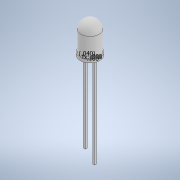
# Autodesk Inventor part: LED
Saved by Autodesk Inventor 2022 (Build 260153000, 153)
## iProperties
Created: 2022-10-09
Part Number: LED
Material: Generic
Document SubType Name: Modeling
Designer: Nick
Density: 1 g/cm^3
Appearance: Default
Author: Nick
Autodesk Inventor part; units mm, degrees
ref_plane "YZ Plane" through (0, 0, 0) normal (1, 0, 0) x (0, 1, 0)
ref_plane "XZ Plane" through (0, 0, 0) normal (0, 1, 0) x (-1, 0, 0)
ref_plane "XY Plane" through (0, 0, 0) normal (0, 0, 1) x (1, 0, 0)
sketch "Sketch1" plane through (0, 0, 0) normal (0, 0, 1) x (1, 0, 0)
  line L0 (0, 0) -> (0, 8.7)
  arc A0 (2.5, 6.2) -> (0, 8.7) centre (0, 6.2) ccw
  line L1 (2.5, 6.2) -> (2.5, 0.7593)
  line L2 (2.5, 0.7593) -> (2.7, 0.7593)
  line L3 (2.7, 0.7593) -> (2.7, 0)
  line L4 (2.7, 0) -> (0, 0)
  dimension "d0" = 5
  dimension "d1" = 0.2
  dimension "d2" = 8.7
  dimension "d3" = 0.7593
  constraints: 10 end point, 3 perpendicular, 2 point on circle, 2 vertical, 1 centre point, 1 point on line, 1 tangent
  measures "d0" diameter of L1 L0
  measures "d1" distance between parallel lines of L1 L3
  measures "d2" distance of L0.start L0.end
  measures "d3" distance of L2.end L3.end
revolve "Revolution1" add sketch "Sketch1" angle 360 about axis through (0, 0, 0) along (0, 1, 0)
sketch "Sketch2" plane through (0, 0, 0) normal (0, -1, 0) x (1, 0, 0)
  line L0 (-1.52, 0.25) -> (-1.02, 0.25)
  line L1 (-1.02, 0.25) -> (-1.02, -0.25)
  line L2 (-1.02, -0.25) -> (-1.52, -0.25)
  line L3 (-1.52, -0.25) -> (-1.52, 0.25)
  line L4 (1.02, 0.25) -> (1.52, 0.25)
  line L5 (1.52, 0.25) -> (1.52, -0.25)
  line L6 (1.52, -0.25) -> (1.02, -0.25)
  line L7 (1.02, -0.25) -> (1.02, 0.25)
  point P0 (0, 0)
  point P1 (1.02, 0)
  dimension "d5" = 2.54
  dimension "d6" = 1.02
  dimension "d7" = 1.02
  dimension "d8" = 0.5
  constraints: 16 end point, 4 parallel, 3 equal length, 2 horizontal, 2 perpendicular, 1 horizontal alignment, 1 midpoint, 1 point on line
  measures "d5" distance between parallel lines of L5 L1
  measures "d6" distance from line of L7 point (0, 0)
  measures "d7" distance from line of L1 point (0, 0)
  measures "d8" distance of L5.end L6.end
extrude "Extrusion1" add sketch "Sketch2" along normal blind 25.4 contours L4 L5 L6 L7
extrude "Extrusion2" add sketch "Sketch2" along normal blind 22.86 contours L0 L1 L2 L3
equation "\"d6\" = d7"
body "Solid1"
